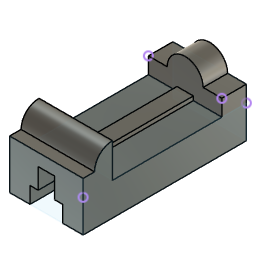
Robocon Task1 b v0 (Autodesk Fusion 360 design; units mm, degrees)
Autodesk Fusion 360 part; units mm, degrees
sketch "Sketch1" plane through (0, 0, 0) normal (0, 0, 1) x (1, 0, 0)
  line L0 (0, 0) -> (0, 100)
  line L1 (0, 100) -> (45, 100)
  line L2 (45, 100) -> (45, 0)
  line L3 (45, 0) -> (0, 0)
  dimension "d1" = 100
  dimension "d2" = 45
  constraint coincident L0.start L3.end
  constraint vertical L0
  constraint perpendicular L0 L1
  constraint perpendicular L1 L2
  constraint perpendicular L0 L3
  measures "d1" distance of L0.start L0.end
  measures "d2" distance of L0.end L1.end
extrude "Extrude1" add sketch "Sketch1" along normal blind 35 makes body 1
extrude "Extrude2" cut 1 faces at (15, 33.3333, 35) along direction (0, 0, -1) blind 15 on bodies 1 bodies 1
sketch "Sketch2" plane through (0, 0, 20) normal (0, 0, 1) x (-1, 0, 0)
  line L0 (-45, -100) -> (0, -100)
  line L1 (0, -100) -> (0, 0)
  line L2 (0, 0) -> (-45, 0)
sketch "Sketch3" plane through (0, 0, 20) normal (0, 0, 1) x (-1, 0, 0)
sketch "Sketch4" plane through (0, 0, 20) normal (0, 0, 1) x (-1, 0, 0)
sketch "Sketch5" plane through (0, 0, 20) normal (0, 0, 1) x (-1, 0, 0)
  line L0 (0, 0) -> (0, -7)
  line L1 (0, -7) -> (-45, -7)
  line L2 (-45, -7) -> (-45, 0)
  line L3 (-45, 0) -> (0, 0)
  constraint coincident L0.start L3.end
  constraint vertical L0
  constraint perpendicular L0 L1
  constraint perpendicular L1 L2
  constraint perpendicular L0 L3
extrude "Extrude3" add sketch "Sketch5" along normal blind 10 bodies 1
sketch "Sketch6" plane through (45, 0, 0) normal (1, 0, 0) x (0, 1, 0)
  line L0 (100, 20) -> (7, 20)
  line L1 (0, 30) -> (0, 0)
  line L2 (0, 0) -> (100, 0)
  line L3 (100, 0) -> (100, 20)
  circle A0 centre (18, 30) radius 11
  line L4 (7, 30) -> (18, 30)
  line L5 (18, 30) -> (18, 20)
  line L6 (18, 30) -> (18, 41)
  line L7 (7, 30) -> (7, 20)
  line L8 (18, 20) -> (18, 30)
  constraint coincident A0 L4.start
  constraint coincident A0.centre L4.end
  constraint horizontal L4
  constraint coincident L0 L5.end
  constraint perpendicular L0 L5
  constraint coincident A0 L6.end
  constraint perpendicular L4 L6
  constraint coincident L0.end L7.end
  constraint tangent A0 L7
extrude "Extrude4" add sketch "Sketch6" against normal blind 45 contours L0 A0 L4 L5 L8 | L0 A0 L7 | A0 L4 L6 bodies 1
sketch "Sketch7" plane through (0, 0, 20) normal (0, 0, 1) x (-1, 0, 0)
  line L0 (-45, -85) -> (0, -85)
  line L1 (0, -85) -> (0, -100)
  line L2 (0, -100) -> (-45, -100)
  line L3 (-45, -100) -> (-45, -85)
  constraint horizontal L0
  constraint perpendicular L0 L1
  constraint perpendicular L1 L2
  constraint perpendicular L0 L3
sketch "Sketch8" plane through (45, 0, 0) normal (1, 0, 0) x (0, 1, 0)
  line L0 (100, 20) -> (18, 20)
  line L1 (18, 20) -> (18, 41)
  arc A0 (18, 41) -> (7, 30) centre (18, 30) ccw
  line L2 (7, 30) -> (0, 30)
  line L3 (0, 30) -> (0, 0)
  line L4 (0, 0) -> (100, 0)
  line L5 (100, 0) -> (100, 20)
extrude "Extrude5" add sketch "Sketch7" along normal blind 10 bodies 1
sketch "Sketch9" plane through (0, 0, 20) normal (0, 0, 1) x (-1, 0, 0)
  line L0 (-45, -85) -> (0, -85)
  line L1 (0, -85) -> (0, -18)
  line L2 (0, -18) -> (-45, -18)
  line L3 (-45, -18) -> (-45, -85)
sketch "Sketch10" plane through (0, 85, 0) normal (0, -1, 0) x (1, 0, 0)
  line L0 (0, 20) -> (45, 20)
  line L1 (45, 20) -> (45, 30)
  line L2 (0, 30) -> (0, 20)
sketch "Sketch11" plane through (0, 100, 0) normal (0, 1, 0) x (-1, 0, 0)
  line L0 (-45, 30) -> (-45, 0)
  line L1 (-45, 0) -> (0, 0)
  line L2 (0, 0) -> (0, 30)
  line L3 (0, 30) -> (-45, 30)
sketch "Sketch12" plane through (0, 100, 0) normal (0, 1, 0) x (-1, 0, 0)
sketch "Sketch13" plane through (45, 0, 0) normal (1, 0, 0) x (0, 1, 0)
sketch "Sketch14" plane through (0, 100, 0) normal (0, 1, 0) x (-1, 0, 0)
sketch "Sketch15" plane through (45, 0, 0) normal (1, 0, 0) x (0, 1, 0)
sketch "Sketch16" plane through (0, 100, 0) normal (0, 1, 0) x (-1, 0, 0)
sketch "Sketch17" plane through (0, 100, 0) normal (0, 1, 0) x (-1, 0, 0)
  line L0 (-45, 30) -> (-22.5, 30)
  line L1 (-22.5, 30) -> (-11.5, 30)
  arc A0 (-11.5, 30) -> (-33.5, 30) centre (-22.5, 30) ccw
  dimension "d17" = 22.5
  dimension "d18" = 22
  constraint horizontal L0
  constraint coincident L0.end L1.start
  constraint parallel L0 L1
  constraint coincident L0 A0.end
  measures "d17" distance of L0.start L0.end
  measures "d18" diameter of A0
extrude "Extrude6" add sketch "Sketch17" against normal blind 15 bodies 1
sketch "Sketch18" plane through (0, 0, 20) normal (0, 0, 1) x (-1, 0, 0)
sketch "Sketch19" plane through (0, 0, 0) normal (0, -1, 0) x (1, 0, 0)
  line L0 (0, 30) -> (0, 0)
  line L1 (0, 0) -> (45, 0)
  line L2 (45, 0) -> (45, 30)
  line L3 (45, 30) -> (0, 30)
sketch "Sketch20" plane through (0, 0, 0) normal (0, -1, 0) x (1, 0, 0)
  line L0 (0, 0) -> (12.5, 0)
  line L1 (45, 0) -> (32.5, 0)
  line L2 (12.5, 0) -> (12.5, 10)
  line L3 (32.5, 0) -> (32.5, 10)
  line L4 (12.5, 10) -> (17.5, 10)
  line L5 (32.5, 10) -> (27.5, 10)
  line L6 (17.5, 10) -> (17.5, 22.5)
  line L7 (27.5, 10) -> (27.5, 22.5)
  line L8 (27.5, 22.5) -> (17.5, 22.5)
  line L9 (12.5, 0) -> (32.5, 0)
  line L10 (17.5, 22.5) -> (17.5, 20)
  line L11 (27.5, 20) -> (17.5, 20)
  line L12 (17.5, 22.5) -> (17.5, 20)
  dimension "d21" = 12.5
  dimension "d22" = 12.5
  dimension "d24" = 10
  dimension "d25" = 5
  dimension "d26" = 5
  dimension "d27" = 12.5
  constraint coincident L0.start origin
  constraint horizontal L0
  constraint horizontal L1
  constraint perpendicular L0 L2
  constraint perpendicular L1 L3
  constraint perpendicular L3 L4
  constraint perpendicular L3 L5
  constraint perpendicular L4 L6
  constraint perpendicular L5 L7
  constraint perpendicular L6 L8
  constraint perpendicular L3 L9
  constraint coincident L6 L10.end
  constraint coincident L7 L11.start
  constraint perpendicular L6 L11
  measures "d21" distance of L0.start L0.end
  measures "d22" distance of L1.start L1.end
  measures "d24" distance of L1.end L3.end
  measures "d25" distance of L2.end L4.end
  measures "d26" distance of L3.end L5.end
  measures "d27" distance of L4.end L6.end
extrude "Extrude7" cut sketch "Sketch20" against normal blind 100 contours L2 L3 L4 L5 L6 L7 L9 L11 bodies 1
sketch "Sketch21" plane through (0, 0, 0) normal (0, -1, 0) x (1, 0, 0)
  line L0 (17.5, 20) -> (17.5, 22.5)
  line L1 (17.5, 22.5) -> (27.5, 22.5)
  line L2 (27.5, 22.5) -> (27.5, 20)
  line L3 (27.5, 20) -> (17.5, 20)
  dimension "d30" = 2.5
  constraint vertical L0
  constraint perpendicular L0 L1
  constraint perpendicular L1 L2
  constraint perpendicular L0 L3
  measures "d30" distance of L0.start L0.end
sketch "Sketch22" plane through (0, 0, 0) normal (0, -1, 0) x (1, 0, 0)
extrude "Extrude8" cut sketch "Sketch21" against normal up to surface (18 mm away) bodies 1
sketch "Sketch23" plane through (0, 18, 0) normal (0, 1, 0) x (-1, 0, 0)
  line L0 (-27.5, 20) -> (-27.5, 22.5)
  line L1 (-27.5, 22.5) -> (-17.5, 22.5)
  line L2 (-17.5, 22.5) -> (-17.5, 20)
  line L3 (-17.5, 20) -> (0, 20)
  line L4 (0, 20) -> (0, 41)
  line L5 (0, 41) -> (-45, 41)
  line L6 (-45, 41) -> (-45, 20)
  line L7 (-45, 20) -> (-27.5, 20)
  line L8 (-27.5, 20) -> (-27.5, 22.5)
  line L9 (-17.5, 22.5) -> (-17.5, 20)
  line L10 (-27.5, 20) -> (-17.5, 20)
  constraint coincident L0.start L7.end
  constraint coincident L0.end L1.start
  constraint coincident L1.end L2.start
  constraint coincident L2.end L3.start
extrude "Extrude9" add sketch "Sketch23" along normal blind 67 separate body contours L0 L1 L2 L8 L9 L10 makes body 2
